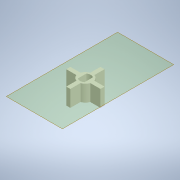
# Autodesk Inventor part: paddle rotor
Saved by Autodesk Inventor 2022 (Build 260153000, 153)
## iProperties
Created: 2022-04-07
Part Number: paddle rotor
Material: Generic
Document SubType Name: Modeling
Designer: efred
Density: 1 g/cm^3
Appearance: Default
Author: efred
Autodesk Inventor part; units mm, degrees
ref_plane "YZ Plane" through (0, 0, 0) normal (1, 0, 0) x (0, 1, 0)
ref_plane "XZ Plane" through (0, 0, 0) normal (0, 1, 0) x (-1, 0, 0)
ref_plane "XY Plane" through (0, 0, 0) normal (0, 0, 1) x (1, 0, 0)
sketch "Sketch1" plane through (0, 0, 0) normal (0, 1, 0) x (-1, 0, 0)
  circle A0 centre (0, 0) radius 3.5
  line L0 (1, -3.3541) -> (-1, -3.3541) construction
  line L1 (-1, -3.3541) -> (-1, -8.3541)
  line L2 (-1, -8.3541) -> (1, -8.3541)
  line L3 (1, -8.3541) -> (1, -3.3541)
  line L4 (0, 0) -> (0, 3.5) construction
  line L5 (8.3541, 1) -> (3.3541, 1)
  line L6 (8.3541, -1) -> (8.3541, 1)
  line L7 (3.3541, -1) -> (8.3541, -1)
  line L8 (-1, 8.3541) -> (-1, 3.3541)
  line L9 (1, 8.3541) -> (-1, 8.3541)
  line L10 (1, 3.3541) -> (1, 8.3541)
  line L11 (-8.3541, -1) -> (-3.3541, -1)
  line L12 (-8.3541, 1) -> (-8.3541, -1)
  line L13 (-3.3541, 1) -> (-8.3541, 1)
  line L14 (3.3541, -1) -> (1, -3.3541) construction
  line L15 (8.3541, -1) -> (1, -8.3541) construction
  dimension "d0" = 7
  dimension "d1" = 2
  dimension "d2" = 5
  dimension "d5" = 360
  dimension "d7" = 3.3292
  dimension "d8" = 10.4003
  dimension "d9" = 3.5355
  constraints: 32 end point, 2 parallel, 2 point on circle, 1 centre point, 1 coincident, 1 horizontal, 1 perpendicular, 1 vertical, 30 other
  measures "d0" diameter of A0
  measures "d1" distance between parallel lines of L1 L3
  measures "d2" distance of L2.end L0.start
  measures "d7" distance of L7.start L0.start
  measures "d8" distance of L6.start L2.end
  measures "d9" distance between parallel lines of L14 L15
extrude "Extrusion1" add sketch "Sketch1" along normal blind 5
sketch "Sketch2" plane through (0, 5, 0) normal (0, 1, 0) x (1, 0, 0)
  circle A0 centre (0, 0) radius 2.6
  line L0 (-1.6, -2.0494) -> (-1.6, 2.0494)
  line L1 (1.6, -2.0494) -> (1.6, 2.0494)
  line L2 (0, 0) -> (0, 2.6) construction
  dimension "d12" = 5.2
  dimension "d13" = 3.2
  constraints: 6 end point, 5 point on circle, 2 parallel, 1 centre point, 1 coincident, 1 vertical, 1 other
  measures "d12" diameter of A0
  measures "d13" distance between parallel lines of L1 L0
extrude "Extrusion2" cut sketch "Sketch2" against normal blind 3 contours L1 A0 L0
sketch "Sketch3" plane through (0, 5, 0) normal (0, 1, 0) x (1, 0, 0)
  line L0 (-1.6, -2.0494) -> (-1.6, 2.0494) projected
  arc A0 (1.6, 2.0494) -> (-1.6, 2.0494) centre (0, 0) ccw projected
  line L1 (1.6, 2.0494) -> (1.6, -2.0494) projected
  arc A1 (-1.6, -2.0494) -> (1.6, -2.0494) centre (0, 0) ccw projected
  arc A2 (-1, 3.3541) -> (-3.3541, 1) centre (0, 0) ccw projected
  line L2 (-3.3541, 1) -> (-8.3541, 1) projected
  line L3 (-8.3541, 1) -> (-8.3541, -1) projected
  line L4 (-8.3541, -1) -> (-3.3541, -1) projected
  arc A3 (-3.3541, -1) -> (-1, -3.3541) centre (0, 0) ccw projected
  line L5 (-1, -3.3541) -> (-1, -8.3541) projected
  line L6 (-1, -8.3541) -> (1, -8.3541) projected
  line L7 (1, -8.3541) -> (1, -3.3541) projected
  arc A4 (1, -3.3541) -> (3.3541, -1) centre (0, 0) ccw projected
  line L8 (3.3541, -1) -> (8.3541, -1) projected
  line L9 (8.3541, -1) -> (8.3541, 1) projected
  line L10 (8.3541, 1) -> (3.3541, 1) projected
  arc A5 (3.3541, 1) -> (1, 3.3541) centre (0, 0) ccw projected
  line L11 (1, 3.3541) -> (1, 8.3541) projected
  line L12 (1, 8.3541) -> (-1, 8.3541) projected
  line L13 (-1, 8.3541) -> (-1, 3.3541) projected
ref_plane "Work Plane1" through (2.25, 8, 0) normal (0, -1, 0) x (-1, 0, 0)
extrude "Extrusion3" add sketch "Sketch3" along normal up to surface (3 mm away)
body "Solid1"
